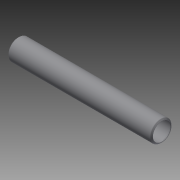
# Autodesk Inventor part: 01R-3.270
Saved by Autodesk Inventor 2015 (Build 190159000, 159)
## iProperties
Category: PARTsolutions
Company: BIMBA
Created: 2015-01-25
Part Number: 01R-3.270
Material: Generic
Catalog Web Link: www.cadenas.de
Description: Tube-Original Line - Standard Air Cylinders
Vendor: BIMBA
Document SubType Name: Standard Catalog Part
Designer: whitaus15
Manufacturer: BIMBA
Mass: 1.54888 g
Surface Area: 62.797 cm^2
Volume: 1.54888 cm^3
Density: 1 g/cm^3
Appearance: PSOLRGB-180-180-180
PSOL_IDENT_0: {$CADENAS_DATA\23d-libs\bimba\bimba\bimba_imperial\bimba_full_line\original_line_cylinders\standard_
PSOL_IDENT_1: air_cylinders\tube.prj},186 {VTYP=3D},{NB=01R-3.270},{LINA=01R-3.270},{NN=Tube},{DATE=08.09.2014 05:
PSOL_IDENT_2: 03:26},{GEOMDATE=18.02.2011 00:00:00},{VERSION=},{LINEID=20},{LINESUBID=-1},{WBVAR=MNT,ACTING,NR,L,F
PSOL_IDENT_3: OURHOLES,SR}  {NB=01R-3.270},{LINA=01R-3.270},{KT=DUMMY},{PN=01R-3.270},{BORE=0.43750000},{BOREPN=01
PSOL_IDENT_4: },{MNT=},{MNTALG='' , 'Front Nose' , 'BF' , 'Front Block' , 'BFT' , 'Front Trunnion'},{ACTING=R},{AC
PSOL_IDENT_5: TINGALG= '' , 'Single Acting' , 'R' , 'Reverse/Double Acting' },{NR=},{NRALG= '' , 'N/A' },{L=3.2700
PSOL_IDENT_6: },{OD=0.4855},{ODN=0.4840},{ODP=0.7380},{ODB=0.0000},{ID=0.4465},{DV=0.00000000},{LV=0.00000000},{LV
PSOL_IDENT_7: 1=0.00000000},{G=0.0200},{FOURHOLES=0},{AA=0.2500},{BB=0.0620},{SR=},{SRALG= 'C' , 'Carbon Steel Rod'
PSOL_IDENT_8: , 'SR' , '303 Stainless Steel Rod' , '' , '303 Stainless Steel Rod'}
NN: Tube
NT: Original Line - Standard Air Cylinders
NB: 01R-3.270
NBSYN: $PN.
LINA: 01R-3.270
BORE: 7/16
BOREPN: 01
MNT: Front Nose
MNTALG: '' , 'Front Nose' , 'BF' , 'Front Block' , 'BFT' , 'Front Trunnion'
ACTING: Reverse/Double Acting
NR: N/A
L: 3.2700
ODN: 0.4840
ODP: 0.7380
ODB: 0.0000
ID: 0.4465
DV: 0.00000000
LV: 0.00000000
LV1: 0.00000000
G: 0.0200
FOURHOLES: 0
AA: 0.2500
BB: 0.0620
SR: 303 Stainless Steel Rod
SUPPLIER: BIMBA
ARTICLENO: 01R-3.270
BOMINFO: 01R-3.270
CREATOR: CADENAS GmbH
Title: 01R-3.270
Author: Cadenas PARTsolutions
Comments: Original Line - Standard Air Cylinders
Autodesk Inventor part; units mm, degrees
sketch "Sketch_1" plane through (0, 0, 0) normal (0, 0, 1) x (1, 0, 0)
  line L0 (83.058, 0) -> (0, 0)
  arc A0 (-0.3964, 5.4846) -> (-0.3964, 5.305) centre (-0.3066, 5.3948) ccw
  line L1 (-0.3964, 5.305) -> (-0.254, 5.1626)
  line L2 (-0.254, 5.1626) -> (0, 5.1626)
  line L3 (0, 5.1626) -> (0.508, 5.6706)
  line L4 (0.508, 5.6706) -> (82.55, 5.6706)
  line L5 (82.55, 5.6706) -> (83.058, 5.1626)
  line L6 (83.058, 5.1626) -> (83.312, 5.1626)
  line L7 (83.312, 5.1626) -> (83.4544, 5.305)
  arc A1 (83.4544, 5.305) -> (83.4544, 5.4846) centre (83.3646, 5.3948) ccw
  line L8 (83.4544, 5.4846) -> (82.9219, 6.0171)
  arc A2 (82.9219, 6.0171) -> (82.5627, 6.1659) centre (82.5627, 5.6578) ccw
  line L9 (82.5627, 6.1659) -> (0.4953, 6.1659)
  arc A3 (0.4953, 6.1659) -> (0.1361, 6.0171) centre (0.4953, 5.6578) ccw
  line L10 (0.1361, 6.0171) -> (-0.3964, 5.4846)
  constraints: 22 end point, 8 point on circle, 4 centre point
revolve "Revolution1" add sketch "Sketch_1" angle 360 about axis through (83.058, 0, 0) along (1, 0, 0)
ref_plane "cp1_XY" through (41.529, 6.1659, 0) normal (1, 0, 0) x (0, 0, -1)
ref_plane "cp1_YZ" through (41.529, 6.1659, 0) normal (0, 0, -1) x (0, 1, 0)
ref_plane "cp1_ZX" through (41.529, 6.1659, 0) normal (0, 1, 0) x (1, 0, 0)
ref_plane "cp2_XY" through (41.529, 0, -6.1659) normal (1, 0, 0) x (0, 0, -1)
ref_plane "cp2_YZ" through (41.529, 0, -6.1659) normal (0, 0, -1) x (0, 1, 0)
ref_plane "cp2_ZX" through (41.529, 0, -6.1659) normal (0, 1, 0) x (1, 0, 0)
ref_plane "cp3_XY" through (41.529, -6.1659, 0) normal (1, 0, 0) x (0, 0, -1)
ref_plane "cp3_YZ" through (41.529, -6.1659, 0) normal (0, 0, -1) x (0, 1, 0)
ref_plane "cp3_ZX" through (41.529, -6.1659, 0) normal (0, 1, 0) x (1, 0, 0)
ref_plane "cp4_XY" through (41.529, 0, 6.1659) normal (1, 0, 0) x (0, 0, -1)
ref_plane "cp4_YZ" through (41.529, 0, 6.1659) normal (0, 0, -1) x (0, 1, 0)
ref_plane "cp4_ZX" through (41.529, 0, 6.1659) normal (0, 1, 0) x (1, 0, 0)
ref_plane "tube_front_XY" through (0, 0, 0) normal (1, 0, 0) x (0, 0, -1)
ref_plane "tube_front_YZ" through (0, 0, 0) normal (0, 0, -1) x (0, 1, 0)
ref_plane "tube_front_ZX" through (0, 0, 0) normal (0, 1, 0) x (1, 0, 0)
ref_plane "tube_rear_XY" through (83.058, 0, 0) normal (1, 0, 0) x (0, 0, -1)
ref_plane "tube_rear_YZ" through (83.058, 0, 0) normal (0, 0, -1) x (0, 1, 0)
ref_plane "tube_rear_ZX" through (83.058, 0, 0) normal (0, 1, 0) x (1, 0, 0)
body "Solid1"
